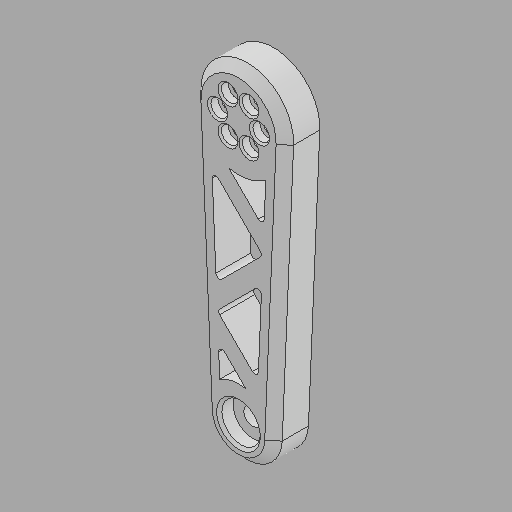
# Autodesk Inventor part: UPPER_LINKAGE_LH
Saved by Autodesk Inventor 2025.2 (Build 292293000, 293)
## iProperties
Created: 2026-05-25
Part Number: UPPER_LINKAGE_LH
Material: Generic
Document SubType Name: Modeling
Designer: Ben
Density: 1 g/cm^3
Appearance: Default
Author: Ben
Autodesk Inventor part; units mm, degrees
ref_plane "YZ Plane" through (0, 0, 0) normal (1, 0, 0) x (0, 1, 0)
ref_plane "XZ Plane" through (0, 0, 0) normal (0, 1, 0) x (-1, 0, 0)
ref_plane "XY Plane" through (0, 0, 0) normal (0, 0, 1) x (1, 0, 0)
sketch "Sketch1" plane through (0, 0, 0) normal (0, 0, 1) x (1, 0, 0)
  circle A0 centre (0, 0) radius 26.5
  circle A1 centre (0, -150) radius 20
  line L0 (-26.4751, -1.1483) -> (-19.9812, -150.8667)
  line L1 (26.4751, -1.1483) -> (19.9812, -150.8667)
  line L2 (-15.5859, -21.432) -> (-10.7412, -133.1291)
  line L3 (15.5859, -21.432) -> (10.7412, -133.1291)
  line L4 (-5.5859, -25.9046) -> (14.5199, -46.0104)
  line L5 (-15.1953, -30.4373) -> (13.932, -59.5646)
  line L6 (-37.1, 0) -> (37.1, 0) projected
  line L7 (13.932, -59.5646) -> (-12.7736, -86.2702)
  line L8 (13.2907, -74.3479) -> (-12.1857, -99.8244)
  line L9 (-12.1857, -99.8244) -> (11.1726, -123.1827)
  line L10 (-11.5445, -114.6078) -> (4.3198, -130.4721)
  point P0 (-26.5, 0)
  point P1 (26.5, 0)
  dimension "d0" = 53
  dimension "d1" = 40
  dimension "d2" = 150
  dimension "d4" = 10
  dimension "d5" = 10
  dimension "d6" = 10
  dimension "d7" = 45
  dimension "d8" = 10
  dimension "d9" = 10
  dimension "d10" = 90
  dimension "d11" = 90
  dimension "d12" = 10
  constraints: 20 end point, 10 point on circle, 8 point on line, 5 parallel, 4 tangent, 2 centre point, 1 coincident, 1 vertical alignment
  measures "d0" diameter of A0
  measures "d1" diameter of A1
  measures "d2" distance of A1.centre point (0, 0)
  measures "d4" distance between parallel lines of L0 L2
  measures "d5" distance between parallel lines of L1 L3
  measures "d6" distance between parallel lines of L5 L4
  measures "d7" angle of L4 L6
  measures "d8" horizontal distance of L2.start L4.start
  measures "d9" distance between parallel lines of L8 L7
  measures "d10" angle of L7 L5
  measures "d11" angle of L9 L8
  measures "d12" distance between parallel lines of L9 L10
extrude "Extrusion1" add sketch "Sketch1" along normal blind 20 contours A0 L6 | A0 L2 A1 L0 | A0 L4 L3 L5 L2 | A0 L6 | A1 | A1 L3 A0 L1 | L7 L3 L8 L2 | L10 L2 L9 L3 A1
sketch "Sketch2" plane through (0, 0, 20) normal (0, 0, 1) x (1, 0, 0)
  line L0 (0, -209.3) -> (0, 65.8) projected
  line L1 (-6, 10.3923) -> (0, 0) construction
  point P0 (6, 10.3923)
  point P1 (-6, -10.3923)
  point P2 (-12, 0)
  point P3 (12, 0)
  point P4 (6, -10.3923)
  dimension "d18" = 12
  dimension "d19" = 12
  dimension "d22" = 360
  constraints: 2 coincident, 2 end point, 1 symmetric about line, 8 other
  measures "d18" distance of point (6, 10.392) L1.start
  measures "d19" distance of L1.start L1.end
hole "Hole1" at (-6, 10.3923, 20) at (-6, -10.3923, 20) at (-12, 0, 20) at (12, 0, 20) at (6, -10.3923, 20) at (6, 10.3923, 20) direction (0, 0, -1) diameter 4.5 end through all counterbore diameter 9.5 counterbore depth 5
fillet "Fillet1" radius 2 8 edges at (-15.1953, -30.4373, 10) (13.932, -59.5646, 10) (14.5199, -46.0104, 10) (-12.7736, -86.2702, 10) (13.2907, -74.3479, 10) (-12.1857, -99.8244, 10) (11.1726, -123.1827, 10) (-11.5445, -114.6078, 10)
chamfer "Chamfer3" distance 1 angle 45 6 edges at (-12, 4.75, 20) (-6, -5.6423, 20) (-6, 15.1423, 20) (6, -5.6423, 20) (6, 15.1423, 20) (12, 4.75, 20)
chamfer "Chamfer2" distance 5 angle 45 4 edges at (23.2282, -76.0075, 20) (0, 26.5, 20) (-23.2282, -76.0075, 20) (0, -170, 20)
sketch "Sketch3" plane through (0, 0, 20) normal (0, 0, 1) x (1, 0, 0)
  arc A0 (-14.9859, -150.65) -> (14.9859, -150.65) centre (0, -150) ccw projected
  point P0 (0, 0)
  constraints: 1 coincident
hole "Hole2" at (0, -150, 20) direction (0, 0, -1) diameter 10 end through all counterbore diameter 22 counterbore depth 8
chamfer "Chamfer4" distance 1.5 angle 45 1 edges at (0, -139, 20)
body "Solid1"
